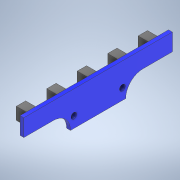
# Autodesk Inventor part: czujnik_podczerwien
Saved by Autodesk Inventor 2022 (Build 260153000, 153)
## iProperties
Created: 2025-05-07
Part Number: czujnik_podczerwien
Material: Ogólny
Document SubType Name: Modeling
Designer: Olga Kowalczyk IB 240875
Density: 1 g/cm^3
Appearance: Domyślna
Author: Olga Kowalczyk IB 240875
Autodesk Inventor part; units mm, degrees
ref_plane "YZ Plane" through (0, 0, 0) normal (1, 0, 0) x (0, 1, 0)
ref_plane "XZ Plane" through (0, 0, 0) normal (0, 1, 0) x (-1, 0, 0)
ref_plane "XY Plane" through (0, 0, 0) normal (0, 0, 1) x (1, 0, 0)
sketch "Szkic1" plane through (0, 0, 0) normal (1, 0, 0) x (0, 1, 0)
  line L0 (9, 0) -> (18, 0)
  line L1 (18, 0) -> (18, -78)
  line L2 (18, -78) -> (9, -78)
  line L3 (0, -53.5) -> (0, -24.5)
  arc A0 (0, -24.5) -> (9, -15.5) centre (0, -15.5) ccw
  arc A1 (9, -62.5) -> (0, -53.5) centre (0, -62.5) ccw
  line L4 (9, 0) -> (9, -15.5)
  line L5 (9, -62.5) -> (9, -78)
  circle A2 centre (5.8, -26.25) radius 1.5
  circle A3 centre (5.8, -51.75) radius 1.5
  line L6 (16.7, -20.55) -> (10.3, -20.55)
  line L7 (10.3, -20.55) -> (10.3, -25.45)
  line L8 (10.3, -25.45) -> (16.7, -25.45)
  line L9 (16.7, -25.45) -> (16.7, -20.55)
  line L10 (16.7, -36.55) -> (10.3, -36.55)
  line L11 (10.3, -36.55) -> (10.3, -41.45)
  line L12 (10.3, -41.45) -> (16.7, -41.45)
  line L13 (16.7, -41.45) -> (16.7, -36.55)
  line L14 (16.7, -52.55) -> (10.3, -52.55)
  line L15 (10.3, -52.55) -> (10.3, -57.45)
  line L16 (10.3, -57.45) -> (16.7, -57.45)
  line L17 (16.7, -57.45) -> (16.7, -52.55)
  line L18 (16.7, -4.55) -> (10.3, -4.55)
  line L19 (10.3, -4.55) -> (10.3, -9.45)
  line L20 (10.3, -9.45) -> (16.7, -9.45)
  line L21 (16.7, -9.45) -> (16.7, -4.55)
  line L22 (16.7, -68.55) -> (10.3, -68.55)
  line L23 (10.3, -68.55) -> (10.3, -73.45)
  line L24 (16.7, -73.45) -> (16.7, -68.55)
  line L25 (16.7, -73.45) -> (10.3, -73.45)
  point P0 (0, 0)
  point P1 (16.7, -71)
  point P2 (16.7, -55)
  point P3 (16.7, -39)
  point P4 (16.7, -23)
  point P5 (16.7, -7)
  dimension "d0" = 9
  dimension "d1" = 78
  dimension "d2" = 15.5
  dimension "d4" = 18
  dimension "d5" = 18
  dimension "d6" = 15.5
  dimension "d7" = 47
  dimension "d8" = 9
  dimension "d9" = 9
  dimension "d10" = 5.8
  dimension "d11" = 26.25
  dimension "d12" = 26.25
  dimension "d13" = 3
  dimension "d14" = 3
  dimension "d15" = 6.4
  dimension "d16" = 4.9
  dimension "d17" = 6.4
  dimension "d18" = 4.9
  dimension "d19" = 6.4
  dimension "d20" = 4.9
  dimension "d21" = 6.4
  dimension "d22" = 4.9
  dimension "d23" = 6.4
  dimension "d24" = 4.9
  dimension "d29" = 16
  dimension "d30" = 16
  dimension "d31" = 16
  dimension "d32" = 16
  dimension "d33" = 4.55
  dimension "d34" = 1.3
  constraints: 52 end point, 11 parallel, 7 horizontal, 7 vertical alignment, 6 perpendicular, 5 midpoint, 4 centre point, 4 coincident, 4 point on circle, 2 point on line, 2 tangent
  measures "d0" distance of L1.end L2.end
  measures "d1" distance of L0.end L1.end
  measures "d2" distance of point (0, 0) point (0, -15.5)
  measures "d4" diameter of A0
  measures "d5" diameter of A1
  measures "d6" vertical distance of L2.end A1.centre
  measures "d7" distance of A1.centre A0.centre
  measures "d8" horizontal distance of L2.end A1.centre
  measures "d9" distance of L0.start L0.end
  measures "d10" distance from line of L3 point (5.8, -51.75)
  measures "d11" distance from line of L2 point (5.8, -51.75)
  measures "d12" distance from line of L0 point (5.8, -26.25)
  measures "d13" diameter of A2
  measures "d14" diameter of A3
  measures "d15" distance of L8.end L7.end
  measures "d16" distance of L7.end L6.end
  measures "d17" distance of L12.end L12.start
  measures "d18" distance of L12.start L10.end
  measures "d19" distance of L16.end L16.start
  measures "d20" distance of L16.start L14.end
  measures "d21" distance of L20.end L20.start
  measures "d22" distance of L20.start L18.end
  measures "d23" distance of L24.start L23.end
  measures "d24" distance of L23.end L22.end
  measures "d29" distance of point (16.7, -23) point (16.7, -7)
  measures "d30" distance of point (16.7, -39) point (16.7, -23)
  measures "d31" distance of point (16.7, -55) point (16.7, -39)
  measures "d32" distance of point (16.7, -71) point (16.7, -55)
  measures "d33" distance between parallel lines of L0 L18
  measures "d34" distance between parallel lines of L1 L21
extrude "Wyciągnięcie proste1" add sketch "Szkic1" along normal blind 2 contours L0 L1 L2 L5 A1 L3 A0 L4 | L9 L8 L7 L6 | L13 L12 L11 L10 | L17 L16 L15 L14 | L21 L20 L19 L18 | L24 L25 L23 L22
extrude "Wyciągnięcie proste2" add sketch "Szkic1" against normal blind 6.5 contours L9 L8 L7 L6 | L13 L12 L11 L10 | L17 L16 L15 L14 | L21 L20 L19 L18 | L24 L25 L23 L22
